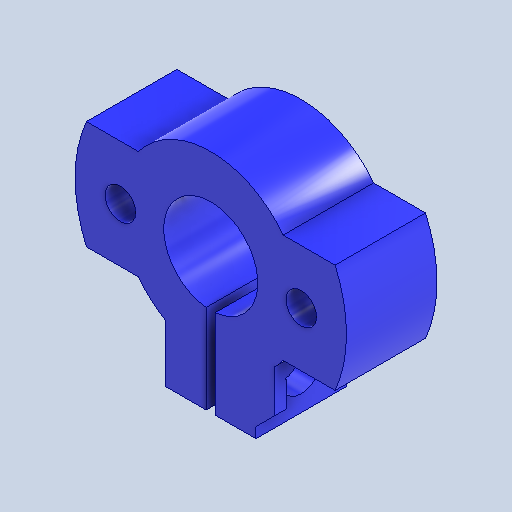
# Autodesk Inventor part: 軸止め
Saved by Autodesk Inventor 2023 (Build 270158000, 158)
## iProperties
Created: 2019-12-20
Part Number: 軸止め
Material: ABS プラスチック
Document SubType Name: Modeling
Designer: Hagihara Yuya
Density: 1.06 g/cm^3
Appearance: 青 - 壁塗料 - 光沢
Mass: 1.99053 g
Surface Area: 15.3185 cm^2
Volume: 1.87786 cm^3
Author: Hagihara Yuya
Autodesk Inventor part; units mm, degrees
ref_plane "YZ Plane" through (0, 0, 0) normal (1, 0, 0) x (0, 1, 0)
ref_plane "XZ Plane" through (0, 0, 0) normal (0, 1, 0) x (-1, 0, 0)
ref_plane "XY Plane" through (0, 0, 0) normal (0, 0, 1) x (1, 0, 0)
sketch "スケッチ1" plane through (0, 0, 0) normal (0, 0, 1) x (1, 0, 0)
  line L0 (0, 0) -> (10, 0)
  line L1 (10, 0) -> (10, 15)
  line L2 (10, 15) -> (0, 15)
  line L3 (0, 15) -> (0, 0)
  circle A0 centre (5, 15) radius 10
  circle A1 centre (5, 15) radius 15
  line L4 (-8.7477, 9) -> (18.7477, 9)
  line L5 (18.7477, 9) -> (18.7477, 21)
  line L6 (18.7477, 21) -> (-8.7477, 21)
  line L7 (-8.7477, 21) -> (-8.7477, 9)
  line L8 (-8.7477, 9) -> (18.7477, 21) construction
  line L9 (18.7477, 9) -> (-8.7477, 21) construction
  point P0 (0, 6.3397)
  point P1 (10, 6.3397)
  point P2 (-8.7477, 9)
  point P3 (-3, 9)
  point P4 (-3, 21)
  point P5 (-8.7477, 21)
  point P6 (13, 21)
  point P7 (13, 9)
  point P8 (18.7477, 9)
  point P9 (10, 9)
  point P10 (0, 9)
  point P11 (-8.7477, 9)
  point P12 (-8.7477, 21)
  point P13 (18.7477, 9)
  point P14 (10, 0.8579)
  point P15 (0, 0.8579)
  point P16 (5, 0)
  dimension "d41" = 30
  dimension "d0" = 15
  dimension "d1" = 20
  dimension "d27" = 10
  dimension "d28" = 5
  dimension "d42" = 12
  constraints: 20 end point, 4 parallel, 3 midpoint, 2 horizontal, 2 perpendicular, 1 centre point, 1 coincident, 3 other
  measures "d0" distance of L2.end L0.start
  measures "d1" diameter of A0
  measures "d27" distance of L1.end L2.end
  measures "d28" distance of A0.centre L2.end
  measures "d42" distance of L4.end L5.end
extrude "押し出し1" add sketch "スケッチ1" along normal blind 10 contours L3 A1 L0 | A1 L1 L0 | A1 L3 A0 L1 | A0 L4 L3 | L3 L4 L1 A0 | L7 L6 A0 L4 | A1 L7 | L1 L4 A0 | L5 A1 | L4 A0 L6 L5 | L4 A0 L6 L1 L2 L3 | L3 L2 L1 L4 | A0 L6
sketch "スケッチ2" plane through (0, 0, 10) normal (0, 0, 1) x (1, 0, 0)
  arc A0 (10, 6.3397) -> (0, 6.3397) centre (5, 15) ccw projected
  point P0 (0, 0)
  point P1 (5, 15)
  constraints: 1 coincident
hole "穴1" at (5, 15, 10) direction (0, 0, -1) diameter 10.4 end through all
sketch "スケッチ3" plane through (0, 0, 10) normal (0, 0, 1) x (1, 0, 0)
  line L0 (0, 0) -> (10, 0) projected
  line L1 (4.5, 0) -> (5.5, 0)
  line L2 (5.5, 0) -> (5.5, 15)
  line L3 (5.5, 15) -> (4.5, 15)
  line L4 (4.5, 15) -> (4.5, 0)
  line L5 (0, 6.3397) -> (0, 0) projected
  circle A0 centre (5, 15) radius 5.2 projected
  point P0 (5, 0)
  point P1 (5, 0)
  dimension "d14" = 1
  constraints: 8 end point, 3 midpoint, 2 coincident, 2 parallel, 1 horizontal, 1 perpendicular, 1 point on line
  measures "d14" distance of L2.end L3.end
extrude "押し出し2" cut sketch "スケッチ3" against normal up to surface (10 mm away) contours L4 A0 L2 L0 | L4 L3 L2 A0 picked at (5.0556, 13.2676)
sketch "スケッチ4" plane through (10, 0, 0) normal (1, 0, 0) x (0, 0, -1)
  circle A0 centre (-5, 4) radius 1.5
  line L0 (0, 0) -> (-10, 0) projected
  line L1 (0, 0) -> (0, 6.3397) projected
  line L2 (-5, 0) -> (-5, 10)
  point P0 (0, 10)
  dimension "d17" = 4
  dimension "d19" = 3
  constraints: 2 end point, 1 centre point, 1 midpoint, 1 point on line, 1 vertical
  measures "d17" distance from line of L0 A0.centre
  measures "d19" diameter of A0
hole "穴2" at (10, 4, 5) direction (-1, 0, 0) diameter 4.4 end through all
sketch "スケッチ7" plane through (10, 0, 0) normal (1, 0, 0) x (0, 0, -1)
  circle A0 centre (-5, 4) radius 2.2 projected
  line L0 (-5, 8.1569) -> (-1.4, 6.0785)
  line L1 (-1.4, 6.0785) -> (-1.4, 1.9215)
  line L2 (-1.4, 1.9215) -> (-5, -0.1569)
  line L3 (-5, -0.1569) -> (-8.6, 1.9215)
  line L4 (-8.6, 1.9215) -> (-8.6, 6.0785)
  line L5 (-8.6, 6.0785) -> (-5, 8.1569)
  line L6 (-10, 9.8241) -> (-10, 0) projected
  line L7 (0, 0) -> (0, 6.3397) projected
  line L8 (-10, 9.8241) -> (0, 9.8241)
  line L9 (0, 9.8241) -> (0, 3.1699)
  line L10 (0, 3.1699) -> (-10, 3.1699)
  line L11 (-10, 3.1699) -> (-10, 9.8241)
  point P0 (-1.4, 3.1699)
  point P1 (0, 6.3397)
  point P2 (-8.6, 3.1699)
  point P3 (-7.0374, 3.1699)
  point P4 (-2.9626, 3.1699)
  dimension "d35" = 7.2
  constraints: 20 end point, 4 coincident, 2 parallel, 1 horizontal, 1 horizontal alignment, 1 midpoint, 1 perpendicular, 13 other
  measures "d35" distance between parallel lines of L0 L3
extrude "押し出し5" add sketch "スケッチ7" along normal blind 2 contours L10 L6 L8 L9 L7 L1 L0 L5 L4
chamfer "面取り1" distance 2 angle 45 2 edges at (10, 3.1699, 9.3) (10, 3.1699, 0.7)
sketch "スケッチ8" plane through (0, 0, 0) normal (0, 0, -1) x (-1, 0, 0)
  circle A0 centre (-5, 15) radius 10 construction
  arc A1 (-4.5, 9.8241) -> (-5.5, 9.8241) centre (-5, 15) ccw construction
  point P0 (0, 0)
  point P1 (5, 15)
  point P2 (-15, 15)
  dimension "d44" = 20
  constraints: 2 horizontal alignment, 2 point on circle, 1 centre point, 1 concentric
  measures "d44" diameter of A0
hole "穴3" at (-5, 15, 0) at (15, 15, 0) direction (0, 0, 1) diameter 3.4 end through all counterbore diameter 5.9 counterbore depth 3
extrude "押し出し7" cut sketch "スケッチ7" along normal through all contours A0 L10 L4 L5 L0 L1
sketch "スケッチ10" plane through (0, 6.3397, 0) normal (-1, 0, 0) x (0, 0, 1)
  circle A0 centre (5, -2.3397) radius 2.2 projected
  circle A1 centre (5, -2.3397) radius 3.7
  point P0 (0, -6.3397)
  dimension "d57" = 7.4
  constraints: 1 centre point, 1 coincident
  measures "d57" diameter of A1
extrude "押し出し8" cut sketch "スケッチ10" along normal blind 10
hole "穴4" at (10, 6.0785, 8.6) at (10, 6.0785, 1.4) at (10, 8.1569, 5) direction (1, 0, 0) diameter 0.3 end through all
equation "\"d28\" = 0.5 * d27"
